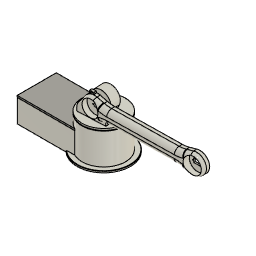
robotic arm project v2 (Autodesk Fusion 360 design; units mm, degrees)
Autodesk Fusion 360 part; units mm, degrees
sketch "Sketch1" plane through (0, 0, 0) normal (0, 0, 1) x (1, 0, 0)
  circle A0 centre (0, 0) radius 66.5
  line L0 (200, 0) -> (-220, 0) construction
  line L1 (-55.1566, 60) -> (-205.1566, 60)
  line L2 (-205.1566, 60) -> (-205.1566, -60)
  line L3 (-205.1566, -60) -> (-55.1566, -60)
  circle A1 centre (0, 0) radius 61.5
  line L4 (-60.1436, 55) -> (-200.1566, 55)
  line L5 (-200.1566, 55) -> (-200.1566, -55)
  line L6 (-200.1566, -55) -> (-60.1436, -55)
  line L7 (-55.1566, 60) -> (-28.6749, 60)
  line L8 (-55.1566, -60) -> (-28.6749, -60)
  line L9 (-60.1436, -55) -> (-37.3798, -55)
  line L10 (-60.1436, 55) -> (-37.3798, 55)
  arc A2 (-55.1566, -60) -> (-55.1566, 60) centre (0, 0) ccw
  dimension "d1" = 133
  dimension "d3" = 150
  dimension "d4" = 120
  dimension "d5" = 150
  dimension "d6" = 123
  dimension "d7" = 5
  dimension "d8" = 5
  dimension "d9" = 5
  dimension "d14" = 15
  constraint coincident A0.centre A1.centre
  constraint horizontal L0
  constraint parallel L0 L1
  constraint perpendicular L1 L2
  constraint perpendicular L2 L3
  constraint symmetric L0 L1 L3
  constraint parallel L1 L4
  constraint perpendicular L0 L5
  constraint perpendicular L5 L6
  constraint coincident A0 L7.end
  constraint parallel L1 L7
  constraint coincident A0 L8.end
  constraint parallel L7 L8
  constraint coincident A0 L9.end
  constraint parallel L8 L9
  constraint coincident A0 L10.end
  constraint parallel L9 L10
  measures "d1" diameter of A0
  measures "d3" distance of L1.start L1.end
  measures "d4" distance of L1.end L2.end
  measures "d5" distance of L2.end L3.end
  measures "d6" diameter of A1
  measures "d7" distance of L1 L4
  measures "d8" distance of L2 L5
  measures "d9" distance of L3 L6
  measures "d14" distance of A0 A2
extrude "Extrude1" add sketch "Sketch1" along normal blind 100 contours A0 makes body 1
extrude "Extrude3" add sketch "Sketch1" along normal blind 5 contours A0 L7 L8 A2 bodies 1
extrude "Extrude4" add sketch "Sketch1" along normal blind 5 contours A0 L4 L5 L6 L9 L10 bodies 1
extrude "Extrude5" add sketch "Sketch1" along normal blind 70 contours A0 L1 L2 L3 L4 L5 L6 L7 L8 L9 L10 bodies 1
fillet "Fillet1" radius 1 1 edges at (81.5, 0, 5) on bodies 1
fillet "Fillet2" radius 1 2 edges at (-205.1566, -60, 35) (-205.1566, 60, 35) on bodies 1
sketch "Sketch2" plane through (0, 0, 70) normal (0, 0, 1) x (-1, 0, 0)
  arc A0 (204.1566, -60) -> (205.1566, -59) centre (204.1566, -59) ccw
  line L0 (205.1566, -59) -> (205.1566, 59)
  arc A1 (205.1566, 59) -> (204.1566, 60) centre (204.1566, 59) ccw
  line L1 (204.1566, 60) -> (28.6749, 60)
  arc A2 (37.3798, 55) -> (28.6749, 60) centre (0, 0) ccw
  line L2 (37.3798, 55) -> (200.1566, 55)
  line L3 (200.1566, 55) -> (200.1566, -55)
  line L4 (200.1566, -55) -> (37.3798, -55)
  arc A3 (28.6749, -60) -> (37.3798, -55) centre (0, 0) ccw
  line L5 (28.6749, -60) -> (204.1566, -60)
  circle A4 centre (198.6566, -53.5) radius 6.5
  circle A5 centre (198.6566, 53.5) radius 6.5
  circle A6 centre (198.6566, -53.5) radius 2
  circle A7 centre (198.6566, 53.5) radius 2
  dimension "d25" = 13
  dimension "d26" = 13
  dimension "d29" = 4
  dimension "d30" = 4
  constraint tangent L0 A4
  constraint tangent L5 A4
  constraint tangent L0 A5
  constraint tangent L1 A5
  constraint concentric A4 A6
  constraint concentric A5 A7
  measures "d25" diameter of A4
  measures "d26" diameter of A5
  measures "d29" diameter of A6
  measures "d30" diameter of A7
extrude "Extrude6" add sketch "Sketch2" against normal up to surface (65 mm away) contours L3 L4 A4 A6 | L3 L4 A6 | L2 L3 A5 A7 | L3 L4 A6 | L2 L3 A7 | L2 L3 A7 picked at (199.416, -48.5705) picked at (199.416, 48.5705) bodies 1
extrude "Extrude7" cut sketch "Sketch2" against normal blind 5 contours L3 L4 A6 | L4 A6 | L3 A6 | L2 L3 A7 | L3 A7 | L2 A7 picked at (199.1968, -54.0205) picked at (199.1771, 54.0402) bodies 1
extrude "Extrude8" add sketch "Sketch1" along normal blind 5 contours A1 bodies 1
sketch "Sketch3" plane through (0, 0, 5) normal (0, 0, 1) x (-1, 0, 0)
  circle A0 centre (0, 0) radius 61.5
  line L0 (15, 20.25) -> (-15, 20.25)
  line L1 (15, -26.9) -> (-15, -26.9)
  line L2 (-15, -26.9) -> (-15, -20.25)
  line L3 (-15, -20.25) -> (15, -20.25)
  line L4 (15, -20.25) -> (15, -26.9)
  line L5 (-15, 20.25) -> (-15, 26.9)
  line L6 (-15, 26.9) -> (15, 26.9)
  line L7 (15, 26.9) -> (15, 20.25)
  line L8 (-30, 0) -> (36.7096, 0) construction
  line L9 (0, -40) -> (0, 50) construction
  dimension "d37" = 30
  dimension "d39" = 30
  dimension "d40" = 6.65
  dimension "d41" = 40.5
  dimension "d43" = 6.65
  constraint horizontal L0
  constraint coincident A0.centre origin
  constraint horizontal L1
  constraint vertical L2
  constraint horizontal L3
  constraint vertical L4
  constraint vertical L5
  constraint horizontal L6
  constraint vertical L7
  constraint parallel L0 L8
  constraint symmetric L0 L3 L8
  constraint coincident L8 A0.centre
  constraint collinear L2 L5
  constraint coincident L0.end L5.start
  constraint perpendicular L6 L9
  constraint coincident A0.centre L9
  constraint symmetric L2 L4 L9
  measures "d37" distance of L1.start L1.end
  measures "d39" distance of L0.start L0.end
  measures "d40" distance of L0.start L6.end
  measures "d41" distance of L0 L3
  measures "d43" distance of L1.end L2.end
extrude "Extrude9" add sketch "Sketch3" along normal blind 85 contours L0 L5 L6 L7 | L1 L2 L3 L4 bodies 1
sketch "Sketch4" plane through (0, 20.25, 0) normal (0, -1, 0) x (1, 0, 0)
  line L0 (-15, 5) -> (15, 5)
  line L1 (15, 5) -> (15, 90)
  line L2 (15, 90) -> (-15, 90)
  line L3 (-15, 90) -> (-15, 5)
  line L4 (-10, 85) -> (10, 85)
  line L5 (10, 85) -> (10, 5)
  line L6 (10, 5) -> (-10, 5)
  line L7 (-10, 5) -> (-10, 85)
  dimension "d47" = 20
  dimension "d48" = 5
  dimension "d49" = 5
  constraint horizontal L4
  constraint vertical L5
  constraint horizontal L6
  constraint vertical L7
  constraint coincident L0 L5.end
  measures "d47" distance of L4.start L4.end
  measures "d48" distance of L2 L4
  measures "d49" distance of L1 L5
extrude "Extrude10" cut sketch "Sketch4" against normal blind 20 contours L0 L4 L5 L6 L7 bodies 1
sketch "Sketch5" plane through (0, -26.9, 0) normal (0, -1, 0) x (1, 0, 0)
  line L0 (-15, 5) -> (15, 5)
  line L1 (15, 5) -> (15, 90)
  line L2 (15, 90) -> (-15, 90)
  line L3 (-15, 90) -> (-15, 5)
  line L4 (-10, 85) -> (10, 85)
  line L5 (10, 85) -> (10, 5)
  line L6 (10, 5) -> (-10, 5)
  line L7 (-10, 5) -> (-10, 85)
  dimension "d52" = 20
  dimension "d53" = 5
  dimension "d54" = 5
  constraint horizontal L4
  constraint vertical L5
  constraint horizontal L6
  constraint vertical L7
  constraint coincident L0 L5.end
  measures "d52" distance of L4.start L4.end
  measures "d53" distance of L2 L4
  measures "d54" distance of L1 L5
extrude "Extrude11" cut sketch "Sketch5" against normal blind 30 contours L0 L4 L5 L6 L7 bodies 1
sketch "Sketch6" plane through (0, 0, 5) normal (0, 0, 1) x (-1, 0, 0)
  line L0 (10, 26.9) -> (15, 26.9)
  line L1 (15, 26.9) -> (15, 20.25)
  line L2 (15, 20.25) -> (10, 20.25)
  line L3 (10, 20.25) -> (10, 26.9)
  line L4 (-10, 26.9) -> (-10, 20.25)
  line L5 (-10, 20.25) -> (-15, 20.25)
  line L6 (-15, 20.25) -> (-15, 26.9)
  line L7 (-15, 26.9) -> (-10, 26.9)
  line L8 (-10, -26.9) -> (-15, -26.9)
  line L9 (-15, -26.9) -> (-15, -20.25)
  line L10 (-15, -20.25) -> (-10, -20.25)
  line L11 (-10, -20.25) -> (-10, -26.9)
  circle A0 centre (0, 0) radius 61.5
  line L12 (10, -26.9) -> (10, -20.25)
  line L13 (10, -20.25) -> (15, -20.25)
  line L14 (15, -20.25) -> (15, -26.9)
  line L15 (15, -26.9) -> (10, -26.9)
  line L16 (15, -26.9) -> (15, -59.6427)
  line L17 (-15, -26.9) -> (-15, -59.6427)
  line L18 (15, 26.9) -> (15, 59.6427)
  line L19 (-15, 26.9) -> (-15, 59.6427)
  line L20 (15, -26.9) -> (-15, -26.9)
  line L21 (15, 26.9) -> (-15, 26.9)
  arc A1 (-15, 59.6427) -> (-15, -59.6427) centre (0, 0) ccw
  arc A2 (15, -59.6427) -> (15, 59.6427) centre (0, 0) ccw
  dimension "d57" = 123
  constraint coincident L14.end L15.start
  constraint coincident A0 L16.end
  constraint perpendicular L15 L16
  constraint coincident L8.end L9.start
  constraint coincident A0 L17.end
  constraint perpendicular L8 L17
  constraint coincident L0.end L1.start
  constraint coincident A0 L18.end
  constraint perpendicular L0 L18
  constraint coincident L6.end L7.start
  constraint coincident A0 L19.end
  constraint perpendicular L7 L19
  constraint coincident A0.centre A1.centre
  constraint concentric A1 A2
  measures "d57" diameter of A1
extrude "Extrude12" cut sketch "Sketch6" against normal through all contours L1 L2 L3 L4 L5 L6 L9 L10 L11 A0 L12 L13 L14 L16 L17 L18 L19 L20 L21 A1 A2 bodies 1
copy_body "Body->Comp1" bodies 1 removing the originals makes body 2 in component "Component"
sketch "Sketch1 (2)" plane through (0, 0, 0) normal (0, 0, 1) x (1, 0, 0) in component "Component'"
  circle A0 centre (0, 0) radius 66.5
  dimension "d59" = 133
  constraint coincident A0.centre origin
  measures "d59" diameter of A0
extrude "Extrude1'" add sketch "Sketch1 (2)" along normal blind 5 separate body makes body 3 in component "Component'"
sketch "Sketch2 (2)" plane through (0, 0, 5) normal (0, 0, 1) x (-1, 0, 0) in component "Component'"
  circle A0 centre (0, 0) radius 66.5
  line L0 (-10, -42.5) -> (-40, -42.5)
  line L1 (-40, -42.5) -> (-40, 42.5)
  line L2 (-40, 42.5) -> (-10, 42.5)
  line L3 (-10, 42.5) -> (-10, -42.5)
  line L4 (66.4951, 0) -> (-66.5, 0) construction
  dimension "d62" = 40
  dimension "d63" = 30
  dimension "d64" = 85
  constraint horizontal L0
  constraint vertical L1
  constraint horizontal L2
  constraint vertical L3
  constraint coincident A0 L4.end
  constraint perpendicular L3 L4
  constraint coincident A0.centre L4
  constraint symmetric L0 L2 L4
  measures "d62" distance of A0.centre L1
  measures "d63" distance of L0.start L0.end
  measures "d64" distance of L0.end L1.end
extrude "Extrude2" add sketch "Sketch2 (2)" along normal blind 20 contours L0 L1 L2 L3 bodies 3 in component "Component'"
sketch "Sketch3 (2)" plane through (40, 0, 0) normal (1, 0, 0) x (0, 1, 0) in component "Component'"
  line L0 (-42.5, 5) -> (42.5, 5)
  line L1 (42.5, 5) -> (42.5, 25)
  line L2 (42.5, 25) -> (-42.5, 25)
  line L3 (-42.5, 25) -> (-42.5, 5)
  line L4 (-42.5, 25) -> (4.3756, 83.5464)
  line L5 (42.5, 25) -> (55.0452, 52.251)
  line L6 (35.0146, 25) -> (49.8894, 53.1001)
  line L7 (8.0872, 80.1793) -> (-34.9854, 25)
  line L8 (35.0146, 25) -> (-34.9854, 25)
  arc A0 (49.8894, 53.1001) -> (8.0872, 80.1793) centre (27.7941, 64.7962) ccw
  arc A1 (55.0452, 52.251) -> (4.3756, 83.5464) centre (27.7941, 64.7962) ccw
  line L9 (35.0146, 25) -> (35.0146, 5)
  line L10 (35.0146, 5) -> (-34.9854, 5)
  line L11 (-34.9854, 5) -> (-34.9854, 25)
  dimension "d67" = 60
  dimension "d68" = 75
  dimension "d69" = 30
  dimension "d78" = 50
  dimension "d79" = 70
  dimension "d80" = 70
  dimension "d85" = 70
  dimension "d86" = 20
  constraint coincident L2.end L3.start
  constraint tangent L4 A1
  constraint coincident L1.end L2.start
  constraint tangent L5 A1
  constraint concentric A0 A1
  constraint coincident L2 L6.start
  constraint coincident L2 L7.end
  constraint parallel L2 L8
  constraint tangent L6 A0
  constraint tangent L7 A0
  constraint perpendicular L8 L9
  constraint perpendicular L9 L10
  measures "d67" diameter of A1
  measures "d68" distance of L2.end L4.end
  measures "d69" distance of L1.end L5.end
  measures "d78" diameter of A0
  measures "d79" distance of L6.start L7.end
  measures "d80" distance of L7.start L7.end
  measures "d85" distance of L9.end L10.end
  measures "d86" distance of L7.end L10.end
extrude "Extrude4'" add sketch "Sketch3 (2)" against normal blind 30 contours L2 L4 L5 L6 L7 A0 A1 bodies 3 in component "Component'"
extrude "Extrude5'" add sketch "Sketch3 (2)" against normal blind 10 contours L2 L6 L7 L8 A0 bodies 3 in component "Component'"
sketch "Sketch7" plane through (10, 0, 0) normal (-1, 0, 0) x (0, -1, 0) in component "Component'"
  line L0 (34.9854, 25) -> (-35.0146, 25)
  line L1 (-35.0146, 25) -> (-49.8894, 53.1001)
  arc A0 (-8.0872, 80.1793) -> (-49.8894, 53.1001) centre (-27.7941, 64.7962) ccw
  line L2 (-8.0872, 80.1793) -> (34.9854, 25)
  line L3 (42.5, 25) -> (-4.3756, 83.5464)
  arc A1 (-4.3756, 83.5464) -> (-55.0452, 52.251) centre (-27.7941, 64.7962) ccw
  line L4 (-55.0452, 52.251) -> (-42.5, 25)
  line L5 (-42.5, 25) -> (-42.5, 5)
  line L6 (-42.5, 5) -> (42.5, 5)
  line L7 (42.5, 5) -> (42.5, 25)
  line L8 (-35.0146, 25) -> (34.9854, 25)
  line L9 (34.9854, 25) -> (34.9854, 5)
  line L10 (34.9854, 5) -> (-35.0146, 5)
  line L11 (-35.0146, 5) -> (-35.0146, 25)
  dimension "d87" = 70
  dimension "d88" = 20
  constraint horizontal L8
  constraint vertical L9
  constraint horizontal L10
  constraint vertical L11
  constraint coincident L0.end L1.start
  measures "d87" distance of L9.end L10.end
  measures "d88" distance of L0.start L9.end
extrude "Extrude6'" cut sketch "Sketch7" against normal blind 20 contours L0 L6 L8 L9 L10 L11 bodies 3 in component "Component'"
fillet "Fillet3" radius 25 1 edges at (20, 35.0146, 25) on bodies 3 in component "Component'"
fillet "Fillet4" radius 30 1 edges at (25, 42.5, 25) on bodies 3 in component "Component'"
fillet "Fillet5" radius 26 1 edges at (25, -42.5, 25) on bodies 3 in component "Component'"
fillet "Fillet6" radius 30 1 edges at (20, -34.9854, 25) on bodies 3 in component "Component'"
sketch "Sketch8" plane through (30, 0, 0) normal (-1, 0, 0) x (0, -1, 0) in component "Component'"
  arc A0 (34.9854, 14.6774) -> (28.6336, 33.1371) centre (4.9854, 14.6774) ccw
  line L0 (28.6336, 33.1371) -> (-8.0872, 80.1793)
  arc A1 (-8.0872, 80.1793) -> (-49.8894, 53.1001) centre (-27.7941, 64.7962) ccw
  line L1 (-49.8894, 53.1001) -> (-37.9194, 30.4874)
  arc A2 (-35.0146, 18.7913) -> (-37.9194, 30.4874) centre (-60.0146, 18.7913) ccw
  line L2 (-35.0146, 18.7913) -> (-35.0146, 5)
  line L3 (-35.0146, 5) -> (34.9854, 5)
  line L4 (34.9854, 5) -> (34.9854, 14.6774)
  line L5 (-33.8205, 58.507) -> (-16.5, 68.507)
  line L6 (-16.5, 68.507) -> (4, 33)
  line L7 (4, 33) -> (-13.3205, 23)
  line L8 (-13.3205, 23) -> (-33.8205, 58.507)
  line L9 (-61.2681, 0) -> (93.7319, 0) construction
  line L10 (0, 0) -> (0, 90) construction
  dimension "d99" = 41
  dimension "d100" = 20
  dimension "d101" = 60
  dimension "d102" = 4
  dimension "d103" = 33
  constraint perpendicular L5 L6
  constraint parallel L5 L7
  constraint parallel L6 L8
  constraint horizontal L9
  constraint coincident L10.start L9
  constraint coincident L10.start origin
  constraint vertical L10
  measures "d99" distance of L5.start L7.end
  measures "d100" distance of L6.end L7.end
  measures "d101" angle of L8 L9
  measures "d102" distance of L6.end L10
  measures "d103" distance of L6.end L9
extrude "Extrude7'" cut sketch "Sketch8" against normal blind 7 contours L5 L6 L7 L8 bodies 3 in component "Component'"
sketch "Sketch1 (3)" plane through (0, 0, 0) normal (0, 0, 1) x (1, 0, 0) in component "Component''"
  circle A0 centre (0, 0) radius 25
  circle A1 centre (0, 300) radius 25
  line L0 (0, -89.8191) -> (0, 380.1809) construction
  line L1 (-28.9006, 291.9528) -> (-22.9341, 270.525)
  line L2 (28.8991, 291.9475) -> (22.9325, 270.5344)
  line L3 (96.2622, 150) -> (-93.7379, 150) construction
  line L4 (106.5165, 259.9912) -> (-113.8098, 260.0095) construction
  line L5 (28.8991, 8.0525) -> (22.9325, 29.4656)
  line L6 (-28.9006, 8.0472) -> (-22.9341, 29.475)
  line L7 (19.9967, 249.061) -> (19.9967, 50.939)
  line L8 (-20.0022, 249.0657) -> (-20.0022, 50.9343)
  arc A2 (-22.9341, 29.475) -> (-20.0022, 50.9343) centre (-100.0022, 50.9343) ccw
  arc A3 (19.9967, 50.939) -> (22.9325, 29.4656) centre (99.9967, 50.939) ccw
  arc A4 (-20.0022, 249.0657) -> (-22.9341, 270.525) centre (-100.0022, 249.0657) ccw
  arc A5 (22.9325, 270.5344) -> (19.9967, 249.061) centre (99.9967, 249.061) ccw
  arc A6 (-28.9006, 8.0472) -> (28.8991, 8.0525) centre (0, 0) ccw
  arc A7 (28.8991, 291.9475) -> (-28.9006, 291.9528) centre (0, 300) ccw
  point P0 (19.9967, 259.9983)
  dimension "d106" = 50
  dimension "d107" = 60
  dimension "d108" = 60
  dimension "d109" = 50
  dimension "d110" = 300
  dimension "d111" = 150
  dimension "d113" = 40
  dimension "d114" = 33.1662
  dimension "d115" = 80
  dimension "d116" = 80
  dimension "d117" = 80
  dimension "d118" = 80
  dimension "d159" = 198.1219
  dimension "d160" = 198.1314
  dimension "d161" = 39.9989
  constraint coincident A0.centre A6.centre
  constraint concentric A1 A7
  constraint vertical L0
  constraint coincident A0.centre L0
  constraint coincident A1.centre L0
  constraint tangent L2 A7
  constraint tangent L1 A7
  constraint coincident P0 L4
  constraint symmetric L1.start L3 L6.start
  constraint symmetric L2.start L3 L5.start
  constraint tangent L8 A2
  constraint tangent L6 A2
  constraint tangent L7 A3
  constraint tangent L5 A3
  constraint tangent L1 A4
  constraint tangent L8 A4
  constraint coincident P0 L7
  constraint coincident P0 L2
  constraint tangent L7 A5
  constraint tangent L2 A5
  constraint vertical L7
  constraint tangent L5 A6
  constraint tangent L6 A6
  measures "d106" diameter of A0
  measures "d107" diameter of A6
  measures "d108" diameter of A7
  measures "d109" diameter of A1
  measures "d110" distance of A0.centre A1.centre
  measures "d111" distance of A0.centre L3
  measures "d113" distance of A1.centre L4
  measures "d114" distance of L2.start P0
  measures "d115" radius of A2
  measures "d116" radius of A3
  measures "d117" radius of A4
  measures "d118" radius of A5
  measures "d159" vertical distance of L7.end L7.start
  measures "d160" distance of L8.end L8.start
  measures "d161" distance of L7 L8
extrude "Extrude1''" add sketch "Sketch1 (3)" along normal blind 25 separate body makes body 4 in component "Component''"
extrude "Extrude2'" add sketch "Sketch1 (3)" along normal blind 5 contours A0 | A1 bodies 4 in component "Component''"
fillet "Fillet1'" radius 15 12 edges at (25.9158, 281.2409, 25) (0.0027, 330, 25) (-25.9173, 281.2389, 25) (-20.7386, 259.895, 25) (-20.0022, 150, 25) (-20.7386, 40.105, 25) (-25.9173, 18.7611, 25) (0.0027, -30, 25) (25.9158, 18.7591, 25) (20.734, 40.1025, 25) (19.9967, 150, 25) (20.734, 259.8975, 25) on bodies 4 in component "Component''"
ref_plane "WorkPlane1" through (0, 30, 0) normal (0, 1, 0) x (0, 0, 1) in component "Component''"
sketch "Sketch2 (3)" plane through (0, 30, 0) normal (0, 1, 0) x (1, 0, 0) in component "Component''"
  line L0 (9, -7) -> (-9, -7)
  line L1 (-9, -7) -> (-9, -17)
  line L2 (-9, -17) -> (9, -17)
  line L3 (9, -17) -> (9, -7)
  line L4 (9, -7) -> (-9, -17) construction
  line L5 (-9, -7) -> (9, -17) construction
  line L6 (0, 0) -> (0, -100) construction
  point P0 (0, -12)
  dimension "d129" = 7
  dimension "d130" = 18
  dimension "d131" = 10
  constraint horizontal L0
  constraint perpendicular L0 L1
  constraint parallel L0 L2
  constraint parallel L1 L3
  constraint coincident L4 P0
  constraint coincident L5 P0
  constraint coincident L6.start origin
  constraint perpendicular L0 L6
  constraint coincident P0 L6
  measures "d129" distance of L0 L6.start
  measures "d130" distance of L1.end L2.end
  measures "d131" distance of L0.start L2.end
sketch "Sketch3 (3)" plane through (0, 0, 5) normal (0, 0, 1) x (-1, 0, 0) in component "Component''"
  circle A0 centre (0, -300) radius 25
  circle A1 centre (0, -300) radius 5
  circle A2 centre (0, -292) radius 1.5
  circle A3 centre (0, -308) radius 1.5
  line L0 (0, -286) -> (0, -318) construction
  dimension "d134" = 10
  dimension "d135" = 3
  dimension "d136" = 3
  dimension "d137" = 8
  dimension "d138" = 8
  constraint concentric A0 A1
  constraint vertical L0
  constraint coincident A0.centre L0
  constraint coincident A2.centre L0
  constraint coincident A3.centre L0
  measures "d134" diameter of A1
  measures "d135" diameter of A2
  measures "d136" diameter of A3
  measures "d137" distance of A0.centre A2.centre
  measures "d138" distance of A0.centre A3.centre
extrude "Extrude4''" cut sketch "Sketch3 (3)" against normal blind 25 contours A1 | A2 | A3 bodies 4 in component "Component''"
sketch "Sketch4 (2)" plane through (0, 0, 5) normal (0, 0, 1) x (-1, 0, 0) in component "Component''"
  circle A0 centre (0, 0) radius 25
  line L0 (6.5, -12) -> (-6.5, -12)
  line L1 (-6.5, -12) -> (-6.5, 12)
  line L2 (-6.5, 12) -> (6.5, 12)
  line L3 (6.5, 12) -> (6.5, -12)
  line L4 (6.5, -12) -> (-6.5, 12) construction
  line L5 (-6.5, -12) -> (6.5, 12) construction
  dimension "d141" = 13
  dimension "d142" = 24
  constraint horizontal L0
  constraint perpendicular L0 L1
  constraint parallel L0 L2
  constraint parallel L1 L3
  constraint coincident L4 A0.centre
  constraint coincident L5 A0.centre
  constraint coincident A0.centre origin
  measures "d141" distance of L1.end L2.end
  measures "d142" distance of L0.end L1.end
extrude "Extrude5''" cut sketch "Sketch4 (2)" against normal blind 60 contours L0 L1 L2 L3 bodies 4 in component "Component''"
sketch "Sketch5 (2)" plane through (0, 0, 5) normal (0, 0, 1) x (-1, 0, 0) in component "Component''"
  line L0 (-6.5, -12) -> (-6.5, 12)
  line L1 (-6.5, 12) -> (6.5, 12)
  line L2 (6.5, 12) -> (6.5, -12)
  line L3 (6.5, -12) -> (-6.5, -12)
  circle A0 centre (0, 0) radius 25
  circle A1 centre (0, -14) radius 1.5
  circle A2 centre (0, 14) radius 1.5
  line L4 (0, -20) -> (0, 19) construction
  dimension "d145" = 3
  dimension "d146" = 3
  dimension "d147" = 14
  dimension "d148" = 14
  constraint perpendicular L3 L4
  constraint coincident A0.centre L4
  constraint coincident A1.centre L4
  constraint coincident A2.centre L4
  measures "d145" diameter of A1
  measures "d146" diameter of A2
  measures "d147" distance of A0.centre A1.centre
  measures "d148" distance of A0.centre A2.centre
extrude "Extrude6''" cut sketch "Sketch5 (2)" against normal blind 20 contours A1 | A2 bodies 4 in component "Component''"
sketch "Sketch6 (2)" plane through (0, 0, 0) normal (1, 0, 0) x (0, 1, 0) in component "Component''"
extrude "Extrude3'" cut sketch "Sketch2 (3)" along normal blind 270 bodies 4 in component "Component''"
ref_plane "WorkPlane2" through (35, 0, 0) normal (1, 0, 0) x (0, 1, 0) in component "Component''"
sketch "Sketch7 (2)" plane through (35, 0, 0) normal (1, 0, 0) x (0, 1, 0) in component "Component''"
  line L0 (302, 9) -> (305, 9)
  line L1 (305, 9) -> (305, 1)
  line L2 (305, 1) -> (302, 1)
  line L3 (302, 1) -> (302, 9)
  line L4 (312, 9) -> (315, 9)
  line L5 (315, 9) -> (315, 1)
  line L6 (315, 1) -> (312, 1)
  line L7 (312, 1) -> (312, 9)
  dimension "d152" = 8
  dimension "d153" = 8
  dimension "d154" = 3
  constraint horizontal L0
  constraint vertical L1
  constraint horizontal L2
  constraint vertical L3
  constraint horizontal L4
  constraint vertical L5
  constraint horizontal L6
  constraint vertical L7
  measures "d152" distance of L4.end L5.end
  measures "d153" distance of L0.start L2.end
  measures "d154" distance of L0.start L0.end
extrude "Extrude7''" add sketch "Sketch7 (2)" along normal up to surface end surface at (28.0026, 310.7636, 3.3333) on bodies 4 bodies 4 in component "Component''"
sketch "Sketch8 (2)" plane through (0, 312, 0) normal (0, -1, 0) x (1, 0, 0) in component "Component''"
  line L0 (27.4955, 9) -> (27.4955, 1)
  line L1 (27.4955, 1) -> (35, 1)
  line L2 (35, 1) -> (35, 9)
  line L3 (35, 9) -> (27.4955, 9)
  line L4 (33, 9) -> (35, 9)
  line L5 (35, 9) -> (35, 1)
  line L6 (35, 1) -> (33, 1)
  line L7 (33, 1) -> (33, 9)
  constraint horizontal L4
  constraint vertical L5
  constraint horizontal L6
  constraint vertical L7
  constraint coincident L1.end L2.start
extrude "Extrude8'" add sketch "Sketch8 (2)" along normal up to surface (7 mm away) contours L1 L2 L3 L4 L5 L6 L7 bodies 4 in component "Component''"
sketch "Sketch9" plane through (37, 0, 0) normal (-1, 0, 0) x (0, -1, 0) in component "Component'"
  line L0 (-13.3205, 23) -> (4, 33)
  line L1 (4, 33) -> (-16.5, 68.507)
  line L2 (-16.5, 68.507) -> (-33.8205, 58.507)
  line L3 (-33.8205, 58.507) -> (-13.3205, 23)
  circle A0 centre (-20, 54) radius 5
  dimension "d166" = 10
  measures "d166" diameter of A0
extrude "Extrude8''" cut sketch "Sketch9" against normal blind 36 contours A0 bodies 3 in component "Component'"
sketch "Sketch1 (4)" plane through (0, 0, 0) normal (0, 0, 1) x (1, 0, 0) in component "Component'''"
  line L0 (10, -20.15) -> (-10, -20.15)
  line L1 (-10, -20.15) -> (-10, 20.15)
  line L2 (-10, 20.15) -> (10, 20.15)
  line L3 (10, 20.15) -> (10, -20.15)
  line L4 (10, -20.15) -> (-10, 20.15) construction
  line L5 (-10, -20.15) -> (10, 20.15) construction
  dimension "d173" = 20
  dimension "d174" = 40.3
  constraint horizontal L0
  constraint perpendicular L0 L1
  constraint parallel L0 L2
  constraint parallel L1 L3
  constraint coincident L4 origin
  constraint coincident L5 origin
  measures "d173" distance of L1.end L2.end
  measures "d174" distance of L0.end L1.end
extrude "Extrude1'''" add sketch "Sketch1 (4)" along normal blind 36.6 separate body makes body 5 in component "Component'''"
sketch "Sketch2 (4)" plane through (0, -20.15, 0) normal (0, -1, 0) x (1, 0, 0) in component "Component'''"
  line L0 (-10, 0) -> (10, 0)
  line L1 (10, 0) -> (10, 36.6)
  line L2 (10, 36.6) -> (-10, 36.6)
  line L3 (-10, 36.6) -> (-10, 0)
  line L4 (-10, 31.6) -> (10, 31.6)
  line L5 (10, 31.6) -> (10, 26.6)
  line L6 (10, 26.6) -> (-10, 26.6)
  line L7 (-10, 26.6) -> (-10, 31.6)
  dimension "d177" = 26.6
  dimension "d178" = 5
  constraint horizontal L4
  constraint vertical L5
  constraint horizontal L6
  constraint vertical L7
  constraint coincident L1 L5.end
  constraint coincident L3 L4.start
  measures "d177" distance of L0 L6
  measures "d178" distance of L4.start L6.end
extrude "Extrude2''" add sketch "Sketch2 (4)" along normal blind 6.65 contours L1 L3 L4 L5 L6 L7 bodies 5 in component "Component'''"
sketch "Sketch3 (4)" plane through (0, 0, 31.6) normal (0, 0, 1) x (-1, 0, 0) in component "Component'''"
  line L0 (10, 20.15) -> (10, 26.8)
  line L1 (10, 26.8) -> (-10, 26.8)
  line L2 (-10, 26.8) -> (-10, 20.15)
  line L3 (0, 0) -> (0, 245.075) construction
  line L4 (-10, 23.475) -> (10, 23.475) construction
  circle A0 centre (-2.5, 23.475) radius 1.75
  circle A1 centre (2.5, 23.475) radius 1.65
  line L5 (-10, 20.15) -> (10, 20.15)
  dimension "d181" = 5
  dimension "d182" = 3.3
  dimension "d183" = 3.5
  constraint coincident L3.start origin
  constraint perpendicular L1 L3
  constraint midpoint L2 L4.start
  constraint midpoint L0 L4.end
  constraint coincident L4 A0.centre
  constraint coincident L4 A1.centre
  constraint symmetric L3 A0.centre A1.centre
  measures "d181" distance of A0.centre A1.centre
  measures "d182" diameter of A1
  measures "d183" diameter of A0
extrude "Extrude3''" cut sketch "Sketch3 (4)" against normal blind 100 contours A0 | A1 bodies 5 in component "Component'''"
mirror "Mirror1" about plane through (0, 0, 0) normal (0, 1, 0) of "Extrude2''", "Extrude3''" in component "Component'''"
sketch "Sketch7 (3)" plane through (10, 0, 0) normal (1, 0, 0) x (0, 1, 0) in component "Component'''"
  line L0 (-20.15, 0) -> (20.15, 0)
  line L1 (20.15, 0) -> (20.15, 26.6)
  line L2 (20.15, 26.6) -> (26.8, 26.6)
  line L3 (26.8, 26.6) -> (26.8, 31.6)
  line L4 (26.8, 31.6) -> (20.15, 31.6)
  line L5 (20.15, 31.6) -> (20.15, 36.6)
  line L6 (20.15, 36.6) -> (-20.15, 36.6)
  line L7 (-20.15, 36.6) -> (-20.15, 31.6)
  line L8 (-20.15, 31.6) -> (-26.8, 31.6)
  line L9 (-26.8, 31.6) -> (-26.8, 26.6)
  line L10 (-26.8, 26.6) -> (-20.15, 26.6)
  line L11 (-20.15, 26.6) -> (-20.15, 0)
  line L12 (-20.15, 34.1) -> (0, 36.6)
  constraint midpoint L7 L12.start
  constraint midpoint L6 L12.end
extrude "Extrude7'''" cut sketch "Sketch7 (3)" against normal blind 27 contours L6 L7 L12 bodies 5 in component "Component'''"
sketch "Sketch8 (3)" plane through (0, 0, 36.6) normal (0, 0, 1) x (-1, 0, 0) in component "Component'''"
  line L0 (10, 0) -> (-10, 0)
  line L1 (-10, 0) -> (-10, -20.15)
  line L2 (-10, -20.15) -> (10, -20.15)
  line L3 (10, -20.15) -> (10, 0)
  circle A0 centre (0, -11) radius 2.5
  line L4 (0, -11) -> (0, 0) construction
  dimension "d199" = 5
  dimension "d200" = 11
  constraint coincident A0.centre L4.start
  constraint coincident L4.end origin
  constraint perpendicular L0 L4
  measures "d199" diameter of A0
  measures "d200" distance of L4.end A0.centre
extrude "Extrude8'''" add sketch "Sketch8 (3)" along normal blind 5 contours A0 bodies 5 in component "Component'''"
sketch "Sketch1 (5)" plane through (0, 0, 0) normal (0, 0, 1) x (1, 0, 0) in component "Component''''"
  line L0 (10, -20.15) -> (-10, -20.15)
  line L1 (-10, -20.15) -> (-10, 20.15)
  line L2 (-10, 20.15) -> (10, 20.15)
  line L3 (10, 20.15) -> (10, -20.15)
  line L4 (10, -20.15) -> (-10, 20.15) construction
  line L5 (-10, -20.15) -> (10, 20.15) construction
  dimension "d173_1" = 20
  dimension "d174_1" = 40.3
  constraint horizontal L0
  constraint perpendicular L0 L1
  constraint parallel L0 L2
  constraint parallel L1 L3
  constraint coincident L4 origin
  constraint coincident L5 origin
  measures "d173_1" distance of L1.end L2.end
  measures "d174_1" distance of L0.end L1.end
extrude "Extrude1''''" add sketch "Sketch1 (5)" along normal blind 36.6 separate body makes body 6 in component "Component''''"
sketch "Sketch2 (5)" plane through (0, -20.15, 0) normal (0, -1, 0) x (1, 0, 0) in component "Component''''"
  line L0 (-10, 0) -> (10, 0)
  line L1 (10, 0) -> (10, 36.6)
  line L2 (10, 36.6) -> (-10, 36.6)
  line L3 (-10, 36.6) -> (-10, 0)
  line L4 (-10, 31.6) -> (10, 31.6)
  line L5 (10, 31.6) -> (10, 26.6)
  line L6 (10, 26.6) -> (-10, 26.6)
  line L7 (-10, 26.6) -> (-10, 31.6)
  dimension "d177_1" = 26.6
  dimension "d178_1" = 5
  constraint horizontal L4
  constraint vertical L5
  constraint horizontal L6
  constraint vertical L7
  constraint coincident L1 L5.end
  constraint coincident L3 L4.start
  measures "d177_1" distance of L0 L6
  measures "d178_1" distance of L4.start L6.end
extrude "Extrude2'''" add sketch "Sketch2 (5)" along normal blind 6.65 contours L1 L3 L4 L5 L6 L7 bodies 6 in component "Component''''"
sketch "Sketch3 (5)" plane through (0, 0, 31.6) normal (0, 0, 1) x (-1, 0, 0) in component "Component''''"
  line L0 (10, 20.15) -> (10, 26.8)
  line L1 (10, 26.8) -> (-10, 26.8)
  line L2 (-10, 26.8) -> (-10, 20.15)
  line L3 (0, 0) -> (0, 245.075) construction
  line L4 (-10, 23.475) -> (10, 23.475) construction
  circle A0 centre (-2.5, 23.475) radius 1.75
  circle A1 centre (2.5, 23.475) radius 1.65
  line L5 (-10, 20.15) -> (10, 20.15)
  dimension "d181_1" = 5
  dimension "d182_1" = 3.3
  dimension "d183_1" = 3.5
  constraint coincident L3.start origin
  constraint perpendicular L1 L3
  constraint midpoint L2 L4.start
  constraint midpoint L0 L4.end
  constraint coincident L4 A0.centre
  constraint coincident L4 A1.centre
  constraint symmetric L3 A0.centre A1.centre
  measures "d181_1" distance of A0.centre A1.centre
  measures "d182_1" diameter of A1
  measures "d183_1" diameter of A0
extrude "Extrude3'''" cut sketch "Sketch3 (5)" against normal blind 100 contours A0 | A1 bodies 6 in component "Component''''"
mirror "Mirror1'" about plane through (0, 0, 0) normal (0, 1, 0) of "Extrude2'''", "Extrude3'''" in component "Component''''"
sketch "Sketch7 (4)" plane through (10, 0, 0) normal (1, 0, 0) x (0, 1, 0) in component "Component''''"
  line L0 (-20.15, 0) -> (20.15, 0)
  line L1 (20.15, 0) -> (20.15, 26.6)
  line L2 (20.15, 26.6) -> (26.8, 26.6)
  line L3 (26.8, 26.6) -> (26.8, 31.6)
  line L4 (26.8, 31.6) -> (20.15, 31.6)
  line L5 (20.15, 31.6) -> (20.15, 36.6)
  line L6 (20.15, 36.6) -> (-20.15, 36.6)
  line L7 (-20.15, 36.6) -> (-20.15, 31.6)
  line L8 (-20.15, 31.6) -> (-26.8, 31.6)
  line L9 (-26.8, 31.6) -> (-26.8, 26.6)
  line L10 (-26.8, 26.6) -> (-20.15, 26.6)
  line L11 (-20.15, 26.6) -> (-20.15, 0)
  line L12 (-20.15, 34.1) -> (0, 36.6)
  constraint midpoint L7 L12.start
  constraint midpoint L6 L12.end
extrude "Extrude7''''" cut sketch "Sketch7 (4)" against normal blind 27 contours L6 L7 L12 bodies 6 in component "Component''''"
sketch "Sketch8 (4)" plane through (0, 0, 36.6) normal (0, 0, 1) x (-1, 0, 0) in component "Component''''"
  line L0 (10, 0) -> (-10, 0)
  line L1 (-10, 0) -> (-10, -20.15)
  line L2 (-10, -20.15) -> (10, -20.15)
  line L3 (10, -20.15) -> (10, 0)
  circle A0 centre (0, -11) radius 2.5
  line L4 (0, -11) -> (0, 0) construction
  dimension "d199_1" = 5
  dimension "d200_1" = 11
  constraint coincident A0.centre L4.start
  constraint coincident L4.end origin
  constraint perpendicular L0 L4
  measures "d199_1" diameter of A0
  measures "d200_1" distance of L4.end A0.centre
extrude "Extrude8''''" add sketch "Sketch8 (4)" along normal blind 5 contours A0 bodies 6 in component "Component''''"
sketch "Sketch1 (6)" plane through (0, 0, 0) normal (0, 0, 1) x (1, 0, 0) in component "Component'''''"
  line L0 (6, -11.5) -> (-6, -11.5)
  line L1 (-6, -11.5) -> (-6, 11.5)
  line L2 (-6, 11.5) -> (6, 11.5)
  line L3 (6, 11.5) -> (6, -11.5)
  line L4 (6, -11.5) -> (-6, 11.5) construction
  line L5 (-6, -11.5) -> (6, 11.5) construction
  dimension "d173_2" = 12
  dimension "d174_2" = 23
  constraint horizontal L0
  constraint perpendicular L0 L1
  constraint parallel L0 L2
  constraint parallel L1 L3
  constraint coincident L4 origin
  constraint coincident L5 origin
  measures "d173_2" distance of L1.end L2.end
  measures "d174_2" distance of L0.end L1.end
extrude "Extrude1'''''" add sketch "Sketch1 (6)" along normal blind 28.5 separate body makes body 7 in component "Component'''''"
sketch "Sketch2 (6)" plane through (0, -11.5, 0) normal (0, -1, 0) x (1, 0, 0) in component "Component'''''"
  line L0 (-6, 0) -> (6, 0)
  line L1 (6, 0) -> (6, 28.5)
  line L2 (6, 28.5) -> (-6, 28.5)
  line L3 (-6, 28.5) -> (-6, 0)
  line L4 (-6, 22.5) -> (6, 22.5)
  line L5 (6, 22.5) -> (6, 19.5)
  line L6 (6, 19.5) -> (-6, 19.5)
  line L7 (-6, 19.5) -> (-6, 22.5)
  dimension "d177_2" = 19.5
  dimension "d178_2" = 3
  constraint horizontal L4
  constraint vertical L5
  constraint horizontal L6
  constraint vertical L7
  constraint coincident L1 L5.end
  constraint coincident L3 L4.start
  measures "d177_2" distance of L0 L6
  measures "d178_2" distance of L4.start L6.end
extrude "Extrude2''''" add sketch "Sketch2 (6)" along normal blind 4.5 contours L1 L3 L4 L5 L6 L7 bodies 7 in component "Component'''''"
sketch "Sketch3 (6)" plane through (0, 0, 22.5) normal (0, 0, 1) x (-1, 0, 0) in component "Component'''''"
  line L0 (6, 11.5) -> (6, 16)
  line L1 (6, 16) -> (-6, 16)
  line L2 (-6, 16) -> (-6, 11.5)
  line L3 (0, 0) -> (0, 15) construction
  line L4 (-6, 13.75) -> (6, 13.75) construction
  line L5 (-6, 11.5) -> (6, 11.5)
  circle A0 centre (0, 13.75) radius 1.5
  dimension "d203" = 3
  constraint coincident L3.start origin
  constraint perpendicular L1 L3
  constraint midpoint L2 L4.start
  constraint midpoint L0 L4.end
  constraint midpoint L4 A0.centre
  measures "d203" diameter of A0
extrude "Extrude9'" cut sketch "Sketch3 (6)" against normal blind 4.5 contours A0 bodies 7 in component "Component'''''"
mirror "Mirror2" about plane through (0, 0, 0) normal (0, 1, 0) of "Extrude2''''", "Extrude9'" in component "Component'''''"
sketch "Sketch9 (2)" plane through (0, 0, 28.5) normal (0, 0, 1) x (-1, 0, 0) in component "Component'''''"
  line L0 (-6, -11.5) -> (6, -11.5)
  line L1 (6, -11.5) -> (6, 11.5)
  line L2 (6, 11.5) -> (-6, 11.5)
  line L3 (-6, 11.5) -> (-6, -11.5)
  circle A0 centre (0, -7) radius 1.5
  dimension "d208" = 3
  measures "d208" diameter of A0
extrude "Extrude10'" add sketch "Sketch9 (2)" along normal blind 2 contours A0 bodies 7 in component "Component'''''"
sketch "Sketch7 (5)" plane through (-95.1366, -141.003, 90) normal (0, 0, 1) x (-1, 0, 0)
  line L0 (-80.1366, -114.103) -> (-110.1366, -114.103)
  line L1 (-110.1366, -114.103) -> (-110.1366, -120.753)
  line L2 (-110.1366, -120.753) -> (-80.1366, -120.753)
  line L3 (-80.1366, -120.753) -> (-80.1366, -114.103)
sketch "Sketch8 (5)" plane through (0, 0, 0) normal (0, 0, 1) x (1, 0, 0)
  line L0 (-28.7746, 59.9523) -> (-205.4795, 59.9523)
  line L1 (-205.4795, 59.9523) -> (-30.4795, 59.9523)
  line L2 (-28.7991, -59.9405) -> (-205.4795, -59.9405)
  line L3 (-205.4795, -59.9405) -> (-205.4795, 59.9523)
  arc A0 (-28.7746, 59.9523) -> (-28.7991, -59.9405) centre (0, 0) ccw
  line L4 (0, 0) -> (-230, 0) construction
  dimension "d211" = 133
  dimension "d213" = 119.9045
  dimension "d215" = 175
  dimension "d216" = 205.4795
  dimension "d217" = 59.9523
  dimension "d218" = 59.9405
  constraint coincident A0.centre L4.start
  constraint horizontal L0
  constraint horizontal L1
  constraint horizontal L2
  constraint vertical L3
  constraint perpendicular L3 L4
  measures "d211" diameter of A0
  measures "d213" distance of L1.end L2.start
  measures "d215" distance of L0.end L1.end
  measures "d216" distance of A0.centre L3
  measures "d217" distance of L1 L4
  measures "d218" distance of L2 L4
extrude "Extrude13" add sketch "Sketch8 (5)" along normal blind 5 separate body makes body 8
copy_body "Body->Comp2" bodies 8 removing the originals makes body 9 in component "Component''''''"
component "Component" placed x (1, 0, 0) y (0, 1, 0) z (0, 0, 1) at (0, 0, 0)
component "Component'" placed x (1, 0, 0) y (0, 1, 0) z (0, 0, 1) at (0, 0, 102)
component "Component''" placed x (0, 0, 1) y (0, -1, 0) z (1, 0, 0) at (43, 320, 156)
component "Component'''" placed x (1, 0, 0) y (0, 1, 0) z (0, 0, 1) at (0, 0, 0)
component "Component''''" placed x (1, 0, 0) y (0, 1, 0) z (0, 0, 1) at (0, 0, 0)
component "Component'''''" placed x (1, 0, 0) y (0, 1, 0) z (0, 0, 1) at (0, 0, 0)
component "Component''''''" placed x (1, 0, 0) y (0, 1, 0) z (0, 0, 1) at (0.3588, -0.0059, 70)
equation "d6 = 133 mm - 10 mm"
equation "d179 = ( 13.3 / 2 ) * 1 mm"
equation "d179_1 = ( 13.3 / 2 ) * 1 mm"
